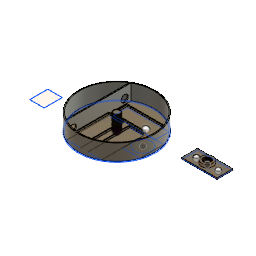
PIR-SensorCase (Autodesk Fusion 360 design; units mm, degrees)
Autodesk Fusion 360 part; units mm, degrees
sketch "Sketch1" plane through (0, 0, 0) normal (0, 1, 0) x (1, 0, 0)
  circle A0 centre (36.25, 0) radius 11.75
  line L0 (24, 16.25) -> (48.5, 16.25)
  line L1 (48.5, 16.25) -> (48.5, -16.25)
  line L2 (48.5, -16.25) -> (24, -16.25)
  line L3 (24, -16.25) -> (24, 16.25)
  line L4 (24, 16.25) -> (48.5, -16.25) construction
  circle A1 centre (0, 0) radius 51.1499
  circle A2 centre (0, 0) radius 52.6499
  line L5 (19.1363, 22.0488) -> (17.75, 22.0488)
  circle A3 centre (0, 0) radius 5
  line L6 (5, 12.8302) -> (24, 12.8302)
  line L7 (24, 12.8302) -> (24, -45.1698)
  line L8 (24, -45.1698) -> (5, -45.1698)
  line L9 (5, -45.1698) -> (5, 12.8302)
  line L10 (-24, 12.8302) -> (-5, 12.8302)
  line L11 (-5, 12.8302) -> (-5, -45.1698)
  line L12 (-5, -45.1698) -> (-24, -45.1698)
  line L13 (-24, -45.1698) -> (-24, 12.8302)
  line L14 (-20.9359, 35.25) -> (37.0641, 35.25)
  line L15 (37.0641, 35.25) -> (37.0641, 16.25)
  line L16 (37.0641, 16.25) -> (-20.9359, 16.25)
  line L17 (-20.9359, 16.25) -> (-20.9359, 35.25)
  dimension "d1" = 23.5
  dimension "d2" = 24.5
  dimension "d3" = 32.5
  dimension "d6" = 1.5
  dimension "d28" = 10
  dimension "d31" = 19
  dimension "d32" = 58
  constraint horizontal L0
  constraint vertical L1
  constraint vertical L3
  constraint midpoint A0.centre L4
  constraint coincident A1.centre A2.centre
  constraint equal L1 L3
  constraint perpendicular L1 L5
  constraint horizontal L6
  constraint vertical L7
  constraint horizontal L8
  constraint vertical L9
  constraint horizontal L10
  constraint vertical L11
  constraint horizontal L12
  constraint vertical L13
  constraint equal L9 L11
  constraint equal L6 L12
  constraint horizontal L14
  constraint vertical L15
  constraint horizontal L16
  constraint vertical L17
  constraint equal L13 L14
  constraint equal L12 L15
  constraint coincident A1 L7.end
  constraint coincident A1 L12.end
  constraint tangent A3 L11
  constraint tangent A3 L9
  constraint coincident L2.end L7
  constraint coincident L1.end A1
  constraint coincident L0.end A1
  constraint coincident A1 L14.end
  constraint coincident L0 L15.end
  measures "d1" diameter of A0
  measures "d2" distance of L0.start L0.end
  measures "d3" distance of L0.start L2.end
  measures "d28" diameter of A3
  measures "d31" distance of L6.start L6.end
  measures "d32" distance of L6.start L8.end
extrude "Extrude2" add sketch "Sketch1" along normal blind 5 contours A0 | L0 L14 L15 L16 L17 | L0 L1 L2 L3 L7 L16 | L3 A1 A3 L6 L9 L10 L11 L13 L14 L16 L17 | L0 A1 L15 | L3 L6 L7 L8 L9 | L1 A1 | L2 A1 L7 | A1 A3 L8 L9 L11 L12 | L10 L11 L12 L13 | A3 makes body 1
extrude "Extrude1" add sketch "Sketch1" along normal blind 23 contours A0 | L0 L14 L15 L16 L17 | L0 L1 L2 L3 L7 L16 | L3 A1 A3 L6 L9 L10 L11 L13 L14 L16 L17 | L0 A1 L15 | L3 L6 L7 L8 L9 | L1 A1 | L2 A1 L7 | A1 A3 L8 L9 L11 L12 | L10 L11 L12 L13 | A3 | A2 bodies 1
fillet "Fillet1" radius 1 1 edges at (-49.0869, 0, 19.039) on bodies 1
shell "Shell1" thickness 1.5 removed faces 1 at (11.5259, 23, 21.5097) on bodies 1
sketch "Sketch2" plane through (0, 1.5, 0) normal (0, 1, 0) x (-1, 0, 0)
  circle A0 centre (0, 0) radius 51.1499
  line L0 (96.5269, -0.9876) -> (76.5269, -0.9876)
  line L1 (76.5269, -0.9876) -> (76.5269, 24.0124)
  line L2 (76.5269, 24.0124) -> (96.5269, 24.0124)
  line L3 (96.5269, 24.0124) -> (96.5269, -0.9876)
  dimension "d11" = 20
  dimension "d12" = 25
  constraint horizontal L0
  constraint vertical L1
  constraint horizontal L2
  constraint vertical L3
  measures "d11" distance of L0.start L0.end
  measures "d12" distance of L0.start L2.end
extrude "Extrude3" cut sketch "Sketch1" along normal through all contours A0 bodies 1
extrude "Extrude4" add sketch "Sketch1" along normal up to surface (23 mm away) contours A3 bodies 1
thread "Thread1" "ISO Metric profile 10.0 M10x1.5 6g" major diameter 9.85 minor diameter 8.141 pitch 1.5 angle 60 modelled right hand crest width 0.1875 on face at (4.9938, 8.6667, -0.2492) crest through (4.925, 1.4063, 0) on bodies 1
sketch "Sketch3" plane through (0, 1.5, 0) normal (0, 1, 0) x (-1, 0, 0)
  line L0 (20.9359, -35.25) -> (-37.0641, -35.25)
  line L1 (20.9359, -16.25) -> (20.9359, -35.25)
  line L2 (-37.0641, -16.25) -> (20.9359, -16.25)
  line L3 (-24, 16.25) -> (-24, -16.25)
  line L4 (-5, -12.8302) -> (-24, -12.8302)
  line L5 (-5, 45.1698) -> (-5, -12.8302)
  line L6 (-24, 45.1698) -> (-5, 45.1698)
  line L7 (5, 45.1698) -> (24, 45.1698)
  line L8 (5, -12.8302) -> (5, 45.1698)
  line L9 (24, -12.8302) -> (5, -12.8302)
  line L10 (24, 45.1698) -> (24, -12.8302)
  line L11 (-37.0641, -35.25) -> (-37.0641, -16.25)
  line L12 (-24, -12.8302) -> (-24, 45.1698)
  line L13 (-38.0641, -15.25) -> (21.9359, -15.25)
  line L14 (21.9359, -15.25) -> (21.9359, -36.25)
  line L15 (21.9359, -36.25) -> (-38.0641, -36.25)
  line L16 (-38.0641, -36.25) -> (-38.0641, -15.25)
  line L17 (-24, 44.1698) -> (-6, 44.1698)
  line L18 (-6, 44.1698) -> (-6, -11.8302)
  line L19 (-6, -11.8302) -> (-24, -11.8302)
  line L20 (25, 46.1698) -> (25, -13.8302)
  line L21 (25, -13.8302) -> (4, -13.8302)
  line L22 (4, -13.8302) -> (4, 46.1698)
  line L23 (4, 46.1698) -> (25, 46.1698)
  line L24 (-24, -16.25) -> (-48.5, -16.25)
  line L25 (-25, -12.8302) -> (-25, 45.1698)
  line L26 (-48.5, 16.25) -> (-24, 16.25)
  circle A0 centre (0, 0) radius 51.1499
  point P0 (-24, -12.8302)
  dimension "d33" = -1
  dimension "d34" = 1
  dimension "d35" = -1
  dimension "d40" = -1
extrude "Extrude7" add sketch "Sketch3" along normal blind 2 contours L12 L25 L26 A0 bodies 1
extrude "Extrude5" add sketch "Sketch3" along normal blind 2 contours L0 L1 L2 L3 L13 L14 L15 A0 | L11 L16 L24 A0 | L15 L16 A0 bodies 1
sketch "Sketch1 (2)" plane through (0, 0, 0) normal (0, 1, 0) x (1, 0, 0) in component "Component"
  line L0 (126.7673, 11.7065) -> (78.774, 11.7065)
  line L1 (78.774, 11.7065) -> (78.774, 33.2608)
  line L2 (78.774, 33.2608) -> (126.7673, 33.2608)
  line L3 (126.7673, 33.2608) -> (126.7673, 11.7065)
  line L4 (126.7673, 11.7065) -> (78.774, 33.2608) construction
  line L5 (78.774, 11.7065) -> (126.7673, 33.2608) construction
  circle A0 centre (102.7707, 22.4836) radius 5 construction
  line L6 (102.7707, 33.2608) -> (102.7707, 11.7065) construction
  point P0 (102.7707, 22.4836)
  point P1 (87.7707, 22.4836)
  point P2 (117.7707, 22.4836)
  dimension "d50" = 10
  dimension "d51" = 30
  constraint perpendicular L0 L1
  constraint parallel L0 L2
  constraint parallel L1 L3
  constraint horizontal L0
  constraint coincident L4 P0
  constraint coincident L5 P0
  constraint coincident P0 A0.centre
  constraint midpoint L2 L6.start
  constraint midpoint L0 L6.end
  constraint symmetric P1 P2 L6
  measures "d50" diameter of A0
  measures "d51" distance of P1 P2
extrude "Extrude1'" add sketch "Sketch1 (2)" along normal blind 2 separate body makes body 2 in component "Component"
sketch "Sketch2 (2)" plane through (0, 2, 0) normal (0, 1, 0) x (-1, 0, 0) in component "Component"
  line L0 (-126.7673, -33.2608) -> (-78.774, -33.2608)
  line L1 (-78.774, -33.2608) -> (-78.774, -11.7065)
  line L2 (-78.774, -11.7065) -> (-126.7673, -11.7065)
  line L3 (-126.7673, -11.7065) -> (-126.7673, -33.2608)
  circle A0 centre (-102.7707, -22.4836) radius 8
  point P0 (-102.7707, -22.4836)
  dimension "d54" = 16
  constraint coincident P0 A0.centre
  measures "d54" diameter of A0
extrude "Extrude2'" add sketch "Sketch2 (2)" along normal blind 4 contours A0 bodies 2 in component "Component"
hole "Hole1" at (102.7707, 6, -22.4836) direction (0, -1, 0) diameter 8.526 end through all bodies 2 in component "Component"
thread "Thread1'" "ISO Metric profile 10.0 M10x1.5 6H" major diameter 10.198 minor diameter 8.526 pitch 1.5 angle 60 modelled right hand crest width 0.1875 on face at (101.7187, 4, -18.3525) crest through (102.7707, 6.8438, -18.2206) on bodies 2 in component "Component"
sketch "Sketch3 (2)" plane through (0, 2, 0) normal (0, 1, 0) x (-1, 0, 0) in component "Component"
  circle A0 centre (-102.7707, -22.4836) radius 8
  line L0 (-126.7673, -33.2608) -> (-78.774, -33.2608)
  line L1 (-78.774, -33.2608) -> (-78.774, -11.7065)
  line L2 (-78.774, -11.7065) -> (-126.7673, -11.7065)
  line L3 (-126.7673, -11.7065) -> (-126.7673, -33.2608)
  point P0 (-87.7707, -22.4836)
  point P1 (-117.7707, -22.4836)
  point P2 (-117.7707, -22.4836)
  point P3 (-87.7707, -22.4836)
  constraint coincident P2 P1
  constraint coincident P3 P0
hole "Hole2" at (87.7707, 2, -22.4836) at (117.7707, 2, -22.4836) direction (0, -1, 0) diameter 3 end through all countersink diameter 6 countersink angle 90 bodies 2 in component "Component"
scale "Scale1" factors (1.03, 1, 1.03) about (102.7707, 6, -26.7466) bodies 2 in component "Component"
extrude "Extrude6" add sketch "Sketch3" along normal blind 2 contours L20 L23 A0 | L20 L21 L22 L23 A0 | L3 L4 L5 L6 L12 L17 L18 L19 bodies 1
sketch "Sketch4" plane through (0, 1.5, 0) normal (0, 1, 0) x (-1, 0, 0)
  circle A0 centre (0, 0) radius 51.1499
  line L0 (25, 44.6241) -> (25, -44.6241)
  line L1 (26.5, 44.6241) -> (26.5, -44.6241)
  point P0 (25, 44.6241)
  point P1 (25, -13.8302)
  dimension "d43" = -1.5
  constraint coincident P0 L0.start
  constraint coincident A0 L0.end
  constraint coincident L0 P1
extrude "Extrude8" add sketch "Sketch4" along normal up to surface (21.5 mm away) contours A0 L0 L1 bodies 1
sketch "Sketch5" plane through (-25, 0, 0) normal (1, 0, 0) x (0, 0, -1)
  line L0 (13.8302, 3.5) -> (13.8302, 1.5)
  line L1 (13.8302, 1.5) -> (44.6241, 1.5)
  line L2 (44.6241, 1.5) -> (44.6241, 23)
  line L3 (44.6241, 23) -> (-44.6241, 23)
  line L4 (-44.6241, 23) -> (-44.6241, 3.5)
  line L5 (-44.6241, 3.5) -> (13.8302, 3.5)
  point P0 (-35.9581, 8.5754)
  point P1 (35.9138, 8.5754)
hole "Hole1'" at (-25, 8.5754, 35.9581) at (-25, 8.5754, -35.9138) direction (-1, 0, 0) diameter 10 depth 2 tip angle 180 bodies 1
component "Component" placed x (1, 0, 0) y (0, 1, 0) z (0, 0, 1) at (0, 0, 0)
equation "d7 = 17 mm + 6 mm"
